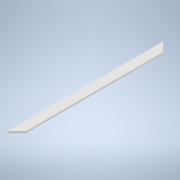
# Autodesk Inventor part: Bridge_Width
Saved by Autodesk Inventor 2020 (Build 240168000, 168)
## iProperties
Created: 2020-07-03
Part Number: Bridge_Width
Material: Generic
Document SubType Name: Modeling
Designer: user
Density: 1 g/cm^3
Appearance: Default
Author: user
Autodesk Inventor part; units mm, degrees
ref_plane "YZ Plane" through (0, 0, 0) normal (1, 0, 0) x (0, 1, 0)
ref_plane "XZ Plane" through (0, 0, 0) normal (0, 1, 0) x (-1, 0, 0)
ref_plane "XY Plane" through (0, 0, 0) normal (0, 0, 1) x (1, 0, 0)
sketch "Sketch1" plane through (0, 0, 0) normal (0, 1, 0) x (-1, 0, 0)
  line L0 (7.8506, 63.4417) -> (2.8506, 63.4417)
  line L1 (2.8506, 63.4417) -> (2.8506, -21.5583)
  line L2 (2.8506, -21.5583) -> (7.8506, -21.5583)
  line L3 (7.8506, -21.5583) -> (7.8506, 63.4417)
  line L4 (7.8506, 63.4417) -> (2.8506, 58.4417)
  line L5 (7.8506, -21.5583) -> (2.8506, -16.5583)
  point P0 (0, 0)
  dimension "d2" = 45
  dimension "d3" = 45
  dimension "d4" = 45
  dimension "d7" = 5
  dimension "d9" = 75
  constraints: 12 end point, 2 parallel, 2 point on line, 1 horizontal, 1 perpendicular
  measures "d2" angle of L4 L0
  measures "d3" angle of L1 L4
  measures "d4" angle of L2 L5
  measures "d7" distance of L1.end L2.end
  measures "d9" distance of L4.end L5.end
extrude "Extrusion1" add sketch "Sketch1" along normal blind 1
extrude "Extrusion2" cut sketch "Sketch1" along normal blind 1 contours L4 L1 L0 | L2 L1 L5
body "Solid1"
